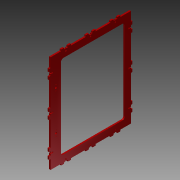
# Autodesk Inventor part: gorna_gt2
Saved by Autodesk Inventor 2013 (Build 170138000, 138)
## iProperties
Created: 2014-01-08
Part Number: gorna_gt2
Material: Generic
Document SubType Name: Modeling
Designer: dzban
Density: 1 g/cm^3
Author: dzban
Autodesk Inventor part; units mm, degrees
ref_plane "YZ Plane" through (0, 0, 0) normal (1, 0, 0) x (0, 1, 0)
ref_plane "XZ Plane" through (0, 0, 0) normal (0, 1, 0) x (-1, 0, 0)
ref_plane "XY Plane" through (0, 0, 0) normal (0, 0, 1) x (1, 0, 0)
sketch "Sketch3" plane through (0, 0, 0) normal (1, 0, 0) x (0, 1, 0)
  line L0 (334.2224, 58.3864) -> (334.2224, 51.3864)
  line L1 (334.2224, 51.3864) -> (340.3224, 51.3864)
  line L2 (340.3224, 51.3864) -> (340.6224, 45.3864)
  line L3 (340.6224, 45.3864) -> (352.4224, 45.3864)
  line L4 (352.4224, 45.3864) -> (352.7224, 51.3864)
  line L5 (352.7224, 51.3864) -> (395.3724, 51.3864)
  line L6 (395.3724, 51.3864) -> (395.3724, 88.9864)
  line L7 (395.3724, 88.9864) -> (401.3724, 89.2864)
  line L8 (401.3724, 89.2864) -> (401.3724, 101.0864)
  line L9 (401.3724, 101.0864) -> (395.3724, 101.3864)
  line L10 (395.3724, 101.3864) -> (395.3724, 107.4864)
  line L11 (395.3724, 107.4864) -> (388.3724, 107.4864)
  line L12 (388.3724, 107.4864) -> (388.3724, 106.2364)
  line L13 (388.3724, 106.2364) -> (386.5724, 106.2364)
  line L14 (386.5724, 106.2364) -> (386.5724, 107.4864)
  line L15 (386.5724, 107.4864) -> (384.7724, 107.4864)
  line L16 (384.7724, 107.4864) -> (384.7724, 110.4864)
  line L17 (384.7724, 110.4864) -> (386.5724, 110.4864)
  line L18 (386.5724, 110.4864) -> (386.5724, 111.7364)
  line L19 (386.5724, 111.7364) -> (388.3724, 111.7364)
  line L20 (388.3724, 111.7364) -> (388.3724, 110.4864)
  line L21 (388.3724, 110.4864) -> (395.3724, 110.4864)
  line L22 (395.3724, 110.4864) -> (395.3724, 116.5864)
  line L23 (395.3724, 116.5864) -> (401.3724, 116.8864)
  line L24 (401.3724, 116.8864) -> (401.3724, 128.6864)
  line L25 (401.3724, 128.6864) -> (395.3724, 128.9864)
  line L26 (395.3724, 128.9864) -> (395.3724, 228.9864)
  line L27 (395.3724, 228.9864) -> (401.3724, 229.2864)
  line L28 (401.3724, 229.2864) -> (401.3724, 241.0864)
  line L29 (401.3724, 241.0864) -> (395.3724, 241.3864)
  line L30 (395.3724, 241.3864) -> (395.3724, 247.4864)
  line L31 (395.3724, 247.4864) -> (388.3724, 247.4864)
  line L32 (388.3724, 247.4864) -> (388.3724, 246.2364)
  line L33 (388.3724, 246.2364) -> (386.5724, 246.2364)
  line L34 (386.5724, 246.2364) -> (386.5724, 247.4864)
  line L35 (386.5724, 247.4864) -> (384.7724, 247.4864)
  line L36 (384.7724, 247.4864) -> (384.7724, 250.4864)
  line L37 (384.7724, 250.4864) -> (386.5724, 250.4864)
  line L38 (386.5724, 250.4864) -> (386.5724, 251.7364)
  line L39 (386.5724, 251.7364) -> (388.3724, 251.7364)
  line L40 (388.3724, 251.7364) -> (388.3724, 250.4864)
  line L41 (388.3724, 250.4864) -> (395.3724, 250.4864)
  line L42 (395.3724, 250.4864) -> (395.3724, 256.5864)
  line L43 (395.3724, 256.5864) -> (401.3724, 256.8864)
  line L44 (401.3724, 256.8864) -> (401.3724, 268.6864)
  line L45 (401.3724, 268.6864) -> (395.3724, 268.9864)
  line L46 (395.3724, 268.9864) -> (395.3724, 368.9864)
  line L47 (395.3724, 368.9864) -> (401.3724, 369.2864)
  line L48 (401.3724, 369.2864) -> (401.3724, 381.0864)
  line L49 (401.3724, 381.0864) -> (395.3724, 381.3864)
  line L50 (395.3724, 381.3864) -> (395.3724, 387.4864)
  line L51 (395.3724, 387.4864) -> (388.3724, 387.4864)
  line L52 (388.3724, 387.4864) -> (388.3724, 386.2364)
  line L53 (388.3724, 386.2364) -> (386.5724, 386.2364)
  line L54 (386.5724, 386.2364) -> (386.5724, 387.4864)
  line L55 (386.5724, 387.4864) -> (384.7724, 387.4864)
  line L56 (384.7724, 387.4864) -> (384.7724, 390.4864)
  line L57 (384.7724, 390.4864) -> (386.5724, 390.4864)
  line L58 (386.5724, 390.4864) -> (386.5724, 391.7364)
  line L59 (386.5724, 391.7364) -> (388.3724, 391.7364)
  line L60 (388.3724, 391.7364) -> (388.3724, 390.4864)
  line L61 (388.3724, 390.4864) -> (395.3724, 390.4864)
  line L62 (395.3724, 390.4864) -> (395.3724, 396.5864)
  line L63 (395.3724, 396.5864) -> (401.3724, 396.8864)
  line L64 (401.3724, 396.8864) -> (401.3724, 408.6864)
  line L65 (401.3724, 408.6864) -> (395.3724, 408.9864)
  line L66 (395.3724, 408.9864) -> (395.3724, 446.5864)
  line L67 (395.3724, 446.5864) -> (352.7224, 446.5864)
  line L68 (352.7224, 446.5864) -> (352.4224, 452.5864)
  line L69 (352.4224, 452.5864) -> (340.6224, 452.5864)
  line L70 (340.6224, 452.5864) -> (340.3224, 446.5864)
  line L71 (340.3224, 446.5864) -> (334.2224, 446.5864)
  line L72 (334.2224, 446.5864) -> (334.2224, 439.5864)
  line L73 (334.2224, 439.5864) -> (335.4724, 439.5864)
  line L74 (335.4724, 439.5864) -> (335.4724, 437.7864)
  line L75 (335.4724, 437.7864) -> (334.2224, 437.7864)
  line L76 (334.2224, 437.7864) -> (334.2224, 435.9864)
  line L77 (334.2224, 435.9864) -> (331.2224, 435.9864)
  line L78 (331.2224, 435.9864) -> (331.2224, 437.7864)
  line L79 (331.2224, 437.7864) -> (329.9724, 437.7864)
  line L80 (329.9724, 437.7864) -> (329.9724, 439.5864)
  line L81 (329.9724, 439.5864) -> (331.2224, 439.5864)
  line L82 (331.2224, 439.5864) -> (331.2224, 446.5864)
  line L83 (331.2224, 446.5864) -> (325.1224, 446.5864)
  line L84 (325.1224, 446.5864) -> (324.8224, 452.5864)
  line L85 (324.8224, 452.5864) -> (313.0224, 452.5864)
  line L86 (313.0224, 452.5864) -> (312.7224, 446.5864)
  line L87 (312.7224, 446.5864) -> (252.7224, 446.5864)
  line L88 (252.7224, 446.5864) -> (252.4224, 452.5864)
  line L89 (252.4224, 452.5864) -> (240.6224, 452.5864)
  line L90 (240.6224, 452.5864) -> (240.3224, 446.5864)
  line L91 (240.3224, 446.5864) -> (234.2224, 446.5864)
  line L92 (234.2224, 446.5864) -> (234.2224, 439.5864)
  line L93 (234.2224, 439.5864) -> (235.4724, 439.5864)
  line L94 (235.4724, 439.5864) -> (235.4724, 437.7864)
  line L95 (235.4724, 437.7864) -> (234.2224, 437.7864)
  line L96 (234.2224, 437.7864) -> (234.2224, 435.9864)
  line L97 (234.2224, 435.9864) -> (231.2224, 435.9864)
  line L98 (231.2224, 435.9864) -> (231.2224, 437.7864)
  line L99 (231.2224, 437.7864) -> (229.9724, 437.7864)
  line L100 (229.9724, 437.7864) -> (229.9724, 439.5864)
  line L101 (229.9724, 439.5864) -> (231.2224, 439.5864)
  line L102 (231.2224, 439.5864) -> (231.2224, 446.5864)
  line L103 (231.2224, 446.5864) -> (225.1224, 446.5864)
  line L104 (225.1224, 446.5864) -> (224.8224, 452.5864)
  line L105 (224.8224, 452.5864) -> (213.0224, 452.5864)
  line L106 (213.0224, 452.5864) -> (212.7224, 446.5864)
  line L107 (212.7224, 446.5864) -> (152.7224, 446.5864)
  line L108 (152.7224, 446.5864) -> (152.4224, 452.5864)
  line L109 (152.4224, 452.5864) -> (140.6224, 452.5864)
  line L110 (140.6224, 452.5864) -> (140.3224, 446.5864)
  line L111 (140.3224, 446.5864) -> (134.2224, 446.5864)
  line L112 (134.2224, 446.5864) -> (134.2224, 439.5864)
  line L113 (134.2224, 439.5864) -> (135.4724, 439.5864)
  line L114 (135.4724, 439.5864) -> (135.4724, 437.7864)
  line L115 (135.4724, 437.7864) -> (134.2224, 437.7864)
  line L116 (134.2224, 437.7864) -> (134.2224, 435.9864)
  line L117 (134.2224, 435.9864) -> (131.2224, 435.9864)
  line L118 (131.2224, 435.9864) -> (131.2224, 437.7864)
  line L119 (131.2224, 437.7864) -> (129.9724, 437.7864)
  line L120 (129.9724, 437.7864) -> (129.9724, 439.5864)
  line L121 (129.9724, 439.5864) -> (131.2224, 439.5864)
  line L122 (131.2224, 439.5864) -> (131.2224, 446.5864)
  line L123 (131.2224, 446.5864) -> (125.1224, 446.5864)
  line L124 (125.1224, 446.5864) -> (124.8224, 452.5864)
  line L125 (124.8224, 452.5864) -> (113.0224, 452.5864)
  line L126 (113.0224, 452.5864) -> (112.7224, 446.5864)
  line L127 (112.7224, 446.5864) -> (70.0724, 446.5864)
  line L128 (70.0724, 446.5864) -> (70.0724, 408.9864)
  line L129 (70.0724, 408.9864) -> (64.0724, 408.6864)
  line L130 (64.0724, 408.6864) -> (64.0724, 396.8864)
  line L131 (64.0724, 396.8864) -> (70.0724, 396.5864)
  line L132 (70.0724, 396.5864) -> (70.0724, 390.4864)
  line L133 (70.0724, 390.4864) -> (77.0724, 390.4864)
  line L134 (77.0724, 390.4864) -> (77.0724, 391.7364)
  line L135 (77.0724, 391.7364) -> (78.8724, 391.7364)
  line L136 (78.8724, 391.7364) -> (78.8724, 390.4864)
  line L137 (78.8724, 390.4864) -> (80.6724, 390.4864)
  line L138 (80.6724, 390.4864) -> (80.6724, 387.4864)
  line L139 (80.6724, 387.4864) -> (78.8724, 387.4864)
  line L140 (78.8724, 387.4864) -> (78.8724, 386.2364)
  line L141 (78.8724, 386.2364) -> (77.0724, 386.2364)
  line L142 (77.0724, 386.2364) -> (77.0724, 387.4864)
  line L143 (77.0724, 387.4864) -> (70.0724, 387.4864)
  line L144 (70.0724, 387.4864) -> (70.0724, 381.3864)
  line L145 (70.0724, 381.3864) -> (64.0724, 381.0864)
  line L146 (64.0724, 381.0864) -> (64.0724, 369.2864)
  line L147 (64.0724, 369.2864) -> (70.0724, 368.9864)
  line L148 (70.0724, 368.9864) -> (70.0724, 268.9864)
  line L149 (70.0724, 268.9864) -> (64.0724, 268.6864)
  line L150 (64.0724, 268.6864) -> (64.0724, 256.8864)
  line L151 (64.0724, 256.8864) -> (70.0724, 256.5864)
  line L152 (70.0724, 256.5864) -> (70.0724, 250.4864)
  line L153 (70.0724, 250.4864) -> (77.0724, 250.4864)
  line L154 (77.0724, 250.4864) -> (77.0724, 251.7364)
  line L155 (77.0724, 251.7364) -> (78.8724, 251.7364)
  line L156 (78.8724, 251.7364) -> (78.8724, 250.4864)
  line L157 (78.8724, 250.4864) -> (80.6724, 250.4864)
  line L158 (80.6724, 250.4864) -> (80.6724, 247.4864)
  line L159 (80.6724, 247.4864) -> (78.8724, 247.4864)
  line L160 (78.8724, 247.4864) -> (78.8724, 246.2364)
  line L161 (78.8724, 246.2364) -> (77.0724, 246.2364)
  line L162 (77.0724, 246.2364) -> (77.0724, 247.4864)
  line L163 (77.0724, 247.4864) -> (70.0724, 247.4864)
  line L164 (70.0724, 247.4864) -> (70.0724, 241.3864)
  line L165 (70.0724, 241.3864) -> (64.0724, 241.0864)
  line L166 (64.0724, 241.0864) -> (64.0724, 229.2864)
  line L167 (64.0724, 229.2864) -> (70.0724, 228.9864)
  line L168 (70.0724, 228.9864) -> (70.0724, 128.9864)
  line L169 (70.0724, 128.9864) -> (64.0724, 128.6864)
  line L170 (64.0724, 128.6864) -> (64.0724, 116.8864)
  line L171 (64.0724, 116.8864) -> (70.0724, 116.5864)
  line L172 (70.0724, 116.5864) -> (70.0724, 110.4864)
  line L173 (70.0724, 110.4864) -> (77.0724, 110.4864)
  line L174 (77.0724, 110.4864) -> (77.0724, 111.7364)
  line L175 (77.0724, 111.7364) -> (78.8724, 111.7364)
  line L176 (78.8724, 111.7364) -> (78.8724, 110.4864)
  line L177 (78.8724, 110.4864) -> (80.6724, 110.4864)
  line L178 (80.6724, 110.4864) -> (80.6724, 107.4864)
  line L179 (80.6724, 107.4864) -> (78.8724, 107.4864)
  line L180 (78.8724, 107.4864) -> (78.8724, 106.2364)
  line L181 (78.8724, 106.2364) -> (77.0724, 106.2364)
  line L182 (77.0724, 106.2364) -> (77.0724, 107.4864)
  line L183 (77.0724, 107.4864) -> (70.0724, 107.4864)
  line L184 (70.0724, 107.4864) -> (70.0724, 101.3864)
  line L185 (70.0724, 101.3864) -> (64.0724, 101.0864)
  line L186 (64.0724, 101.0864) -> (64.0724, 89.2864)
  line L187 (64.0724, 89.2864) -> (70.0724, 88.9864)
  line L188 (70.0724, 88.9864) -> (70.0724, 51.3864)
  line L189 (70.0724, 51.3864) -> (112.7224, 51.3864)
  line L190 (112.7224, 51.3864) -> (113.0224, 45.3864)
  line L191 (113.0224, 45.3864) -> (124.8224, 45.3864)
  line L192 (124.8224, 45.3864) -> (125.1224, 51.3864)
  line L193 (125.1224, 51.3864) -> (131.2224, 51.3864)
  line L194 (131.2224, 51.3864) -> (131.2224, 58.3864)
  line L195 (131.2224, 58.3864) -> (129.9724, 58.3864)
  line L196 (129.9724, 58.3864) -> (129.9724, 60.1864)
  line L197 (129.9724, 60.1864) -> (131.2224, 60.1864)
  line L198 (131.2224, 60.1864) -> (131.2224, 61.9864)
  line L199 (131.2224, 61.9864) -> (134.2224, 61.9864)
  line L200 (134.2224, 61.9864) -> (134.2224, 60.1864)
  line L201 (134.2224, 60.1864) -> (135.4724, 60.1864)
  line L202 (135.4724, 60.1864) -> (135.4724, 58.3864)
  line L203 (135.4724, 58.3864) -> (134.2224, 58.3864)
  line L204 (134.2224, 58.3864) -> (134.2224, 51.3864)
  line L205 (134.2224, 51.3864) -> (140.3224, 51.3864)
  line L206 (140.3224, 51.3864) -> (140.6224, 45.3864)
  line L207 (140.6224, 45.3864) -> (152.4224, 45.3864)
  line L208 (152.4224, 45.3864) -> (152.7224, 51.3864)
  line L209 (152.7224, 51.3864) -> (212.7224, 51.3864)
  line L210 (212.7224, 51.3864) -> (213.0224, 45.3864)
  line L211 (213.0224, 45.3864) -> (224.8224, 45.3864)
  line L212 (224.8224, 45.3864) -> (225.1224, 51.3864)
  line L213 (225.1224, 51.3864) -> (231.2224, 51.3864)
  line L214 (231.2224, 51.3864) -> (231.2224, 58.3864)
  line L215 (231.2224, 58.3864) -> (229.9724, 58.3864)
  line L216 (229.9724, 58.3864) -> (229.9724, 60.1864)
  line L217 (229.9724, 60.1864) -> (231.2224, 60.1864)
  line L218 (231.2224, 60.1864) -> (231.2224, 61.9864)
  line L219 (231.2224, 61.9864) -> (234.2224, 61.9864)
  line L220 (234.2224, 61.9864) -> (234.2224, 60.1864)
  line L221 (234.2224, 60.1864) -> (235.4724, 60.1864)
  line L222 (235.4724, 60.1864) -> (235.4724, 58.3864)
  line L223 (235.4724, 58.3864) -> (234.2224, 58.3864)
  line L224 (234.2224, 58.3864) -> (234.2224, 51.3864)
  line L225 (234.2224, 51.3864) -> (240.3224, 51.3864)
  line L226 (240.3224, 51.3864) -> (240.6224, 45.3864)
  line L227 (240.6224, 45.3864) -> (252.4224, 45.3864)
  line L228 (252.4224, 45.3864) -> (252.7224, 51.3864)
  line L229 (252.7224, 51.3864) -> (312.7224, 51.3864)
  line L230 (312.7224, 51.3864) -> (313.0224, 45.3864)
  line L231 (313.0224, 45.3864) -> (324.8224, 45.3864)
  line L232 (324.8224, 45.3864) -> (325.1224, 51.3864)
  line L233 (325.1224, 51.3864) -> (331.2224, 51.3864)
  line L234 (331.2224, 51.3864) -> (331.2224, 58.3864)
  line L235 (331.2224, 58.3864) -> (329.9724, 58.3864)
  line L236 (329.9724, 58.3864) -> (329.9724, 60.1864)
  line L237 (329.9724, 60.1864) -> (331.2224, 60.1864)
  line L238 (331.2224, 60.1864) -> (331.2224, 61.9864)
  line L239 (331.2224, 61.9864) -> (334.2224, 61.9864)
  line L240 (334.2224, 61.9864) -> (334.2224, 60.1864)
  line L241 (334.2224, 60.1864) -> (335.4724, 60.1864)
  line L242 (335.4724, 60.1864) -> (335.4724, 58.3864)
  line L243 (335.4724, 58.3864) -> (334.2224, 58.3864)
  arc A0 (371.3724, 408.5864) -> (361.3724, 418.5864) centre (361.3724, 408.5864) ccw
  line L244 (371.3724, 408.5864) -> (371.3724, 89.3864)
  arc A1 (361.3724, 79.3864) -> (371.3724, 89.3864) centre (361.3724, 89.3864) ccw
  line L245 (361.3724, 79.3864) -> (122.0724, 79.3864)
  arc A2 (112.0724, 89.3864) -> (122.0724, 79.3864) centre (122.0724, 89.3864) ccw
  line L246 (112.0724, 89.3864) -> (112.0724, 408.5864)
  arc A3 (122.0724, 418.5864) -> (112.0724, 408.5864) centre (122.0724, 408.5864) ccw
  line L247 (122.0724, 418.5864) -> (361.3724, 418.5864)
  circle A4 centre (92.0724, 328.9864) radius 3.95
  circle A5 centre (92.0724, 168.9864) radius 3.95
  circle A6 centre (92.0724, 157.9864) radius 1.5
  circle A7 centre (92.0724, 317.9864) radius 1.5
  circle A8 centre (92.0724, 339.9864) radius 1.5
  circle A9 centre (92.0724, 179.9864) radius 1.5
  point P0 (0, 0)
  dimension "d59" = 51.3865
  dimension "d60" = 70.0724
  dimension "d63" = 395.2
  dimension "d64" = 325.3
  dimension "d65" = 6
  dimension "d66" = 6
  dimension "d67" = 6
  dimension "d68" = 6
  dimension "d69" = 7
  dimension "d70" = 1.8
  dimension "d71" = 1.8
  dimension "d72" = 3
  dimension "d73" = 1.25
  dimension "d74" = 1.25
  dimension "d76" = 12.4
  dimension "d77" = 6.1
  dimension "d78" = 11.8
  dimension "d79" = 0.3
  dimension "d80" = 6.1
  dimension "d81" = 12.4
  dimension "d82" = 100
  dimension "d83" = 6.1
  dimension "d84" = 12.4
  dimension "d85" = 3
  dimension "d86" = 6.1
  dimension "d87" = 12.4
  dimension "d88" = 1.25
  dimension "d89" = 1.25
  dimension "d90" = 100
  dimension "d91" = 6.1
  dimension "d92" = 12.4
  dimension "d93" = 6.1
  dimension "d94" = 12.4
  dimension "d95" = 3
  dimension "d96" = 1.25
  dimension "d97" = 1.25
  dimension "d98" = 10.6
  dimension "d99" = 1.8
  dimension "d100" = 1.8
  dimension "d101" = 28
  dimension "d102" = 42
  dimension "d103" = 24
  dimension "d104" = 28
  dimension "d105" = 10
  dimension "d108" = 7.9
  dimension "d109" = 3
  dimension "d110" = 11
  dimension "d111" = 11
  dimension "d112" = 78.5
  dimension "d113" = 78.5
  dimension "d114" = 22
  dimension "d115" = 10.6
  dimension "d116" = 1.8
  dimension "d117" = 1.8
  dimension "d119" = 6.1
  dimension "d120" = 12.4
  dimension "d121" = 3
  dimension "d122" = 1.25
  dimension "d123" = 1.25
  dimension "d124" = 6.1
  dimension "d125" = 12.4
  dimension "d126" = 140
  dimension "d127" = 6.1
  dimension "d128" = 12.4
  constraints: 496 end point, 196 parallel, 153 collinear, 48 perpendicular, 17 vertical alignment, 12 horizontal alignment, 10 centre point, 8 point on circle, 8 tangent, 7 equal radius, 1 horizontal
  measures "d59" distance from line of L189 point (0, 0)
  measures "d60" distance from line of L188 point (0, 0)
  measures "d63" distance between parallel lines of L127 L189
  measures "d64" distance between parallel lines of L66 L128
  measures "d65" distance between parallel lines of L148 L146
  measures "d66" distance between parallel lines of L125 L127
  measures "d67" distance between parallel lines of L189 L191
  measures "d68" distance between parallel lines of L6 L8
  measures "d69" distance between parallel lines of L195 L193
  measures "d70" distance between parallel lines of L197 L195
  measures "d71" distance between parallel lines of L199 L197
  measures "d72" distance between parallel lines of L204 L194
  measures "d73" distance between parallel lines of L196 L194
  measures "d74" distance between parallel lines of L202 L204
  measures "d76" distance of L192.end L189.end
  measures "d77" distance of L192.end L193.end
  measures "d78" distance of L190.end L191.end
  measures "d79" horizontal distance of L189.end L190.end
  measures "d80" distance of L204.end L205.end
  measures "d81" distance of L208.end L205.end
  measures "d82" distance between parallel lines of L214 L194
  measures "d83" distance of L212.end L213.end
  measures "d84" distance of L209.end L212.end
  measures "d85" distance between parallel lines of L224 L214
  measures "d86" distance of L224.end L225.end
  measures "d87" distance of L228.end L225.end
  measures "d88" distance between parallel lines of L216 L214
  measures "d89" distance between parallel lines of L222 L224
  measures "d90" distance between parallel lines of L234 L214
  measures "d91" distance of L232.end L233.end
  measures "d92" distance of L229.end L232.end
  measures "d93" distance of L0.end L1.end
  measures "d94" distance of L4.end L1.end
  measures "d95" distance between parallel lines of L0 L234
  measures "d96" distance between parallel lines of L242 L0
  measures "d97" distance between parallel lines of L236 L234
  measures "d98" distance between parallel lines of L123 L117
  measures "d99" distance between parallel lines of L119 L117
  measures "d100" distance between parallel lines of L121 L119
  measures "d101" distance between parallel lines of L209 L245
  measures "d102" distance between parallel lines of L246 L168
  measures "d103" distance between parallel lines of L244 L26
  measures "d104" distance between parallel lines of L247 L107
  measures "d105" radius of A3
  measures "d108" diameter of A4
  measures "d109" diameter of A8
  measures "d110" distance of A4.centre A8.centre
  measures "d111" distance of A7.centre A4.centre
  measures "d112" distance from line of L153 A4.centre
  measures "d113" distance from line of A5.centre L163
  measures "d114" distance from line of A4.centre L148
  measures "d115" distance between parallel lines of L62 L56
  measures "d116" distance between parallel lines of L58 L56
  measures "d117" distance between parallel lines of L60 L58
  measures "d119" distance of L61.end L62.end
  measures "d120" distance of L65.end L62.end
  measures "d121" distance between parallel lines of L61 L51
  measures "d122" distance between parallel lines of L59 L61
  measures "d123" distance between parallel lines of L51 L53
  measures "d124" distance of L49.end L50.end
  measures "d125" distance of L49.end L46.end
  measures "d126" distance between parallel lines of L41 L61
  measures "d127" distance of L41.end L42.end
  measures "d128" distance of L45.end L42.end
extrude "Extrusion2" add sketch "Sketch3" along normal blind 6
sketch "Sketch4" plane through (0, 0, 0) normal (-1, 0, 0) x (0, 0, 1)
  line L0 (51.3864, 231.2224) -> (58.3864, 231.2224) projected
  circle A0 centre (444.7864, 232.7224) radius 3.1
  line L1 (446.5864, 240.3224) -> (446.5864, 234.2224) projected
  point P0 (0, 0)
  dimension "d151" = 6.2
  dimension "d153" = 1.5
  dimension "d156" = 1.8
  constraints: 1 centre point
  measures "d151" diameter of A0
  measures "d153" distance from line of A0.centre L0
  measures "d156" distance from line of L1 A0.centre
extrude "Extrusion3" cut sketch "Sketch4" against normal blind 10
body "Solid2"
